Autodesk Fusion 360 part; units mm, degrees
(part 2 of 21)
sketch "Schizzo2" plane through (0, 0, 0) normal (0, 0, 1) x (1, 0, 0) in component "Spur Gear (12 teeth)"
  spline S0 degree 5 poles (5.5783, -0.8192) (5.5823, -0.8197) (5.5902, -0.8208) (5.6021, -0.8219) (5.6181, -0.8228) (5.6381, -0.8229) (5.6583, -0.8223) (5.6784, -0.8212) (5.6986, -0.8199) (5.7188, -0.8184) (5.7391, -0.8168) (5.7593, -0.8149) (5.7796, -0.8127) (5.7999, -0.8102) (5.8203, -0.8073) (5.8406, -0.8041) (5.861, -0.8006) (5.8814, -0.7969) (5.9018, -0.793) (5.9222, -0.7888) (5.9426, -0.7845) (5.9631, -0.7799) (5.9835, -0.7752) (6.0039, -0.7702) (6.0244, -0.765) (6.0448, -0.7596) (6.0653, -0.7539) (6.0857, -0.7481) (6.1061, -0.7421) (6.1266, -0.7359) (6.147, -0.7295) (6.1675, -0.7229) (6.1879, -0.7161) (6.2083, -0.7092) (6.2288, -0.7021) (6.2492, -0.6947) (6.2696, -0.6873) (6.29, -0.6796) (6.3104, -0.6717) (6.3308, -0.6637) (6.3512, -0.6555) (6.3715, -0.6472) (6.3919, -0.6387) (6.4122, -0.63) (6.4325, -0.6211) (6.4528, -0.6121) (6.4731, -0.6029) (6.4934, -0.5936) (6.5137, -0.5841) (6.5339, -0.5744) (6.5541, -0.5646) (6.5743, -0.5546) (6.5945, -0.5445) (6.6147, -0.5342) (6.6348, -0.5238) (6.655, -0.5132) (6.6751, -0.5024) (6.6951, -0.4915) (6.7152, -0.4805) (6.7352, -0.4693) (6.7552, -0.4579) (6.7752, -0.4464) (6.7952, -0.4348) (6.8151, -0.423) (6.835, -0.4111) (6.8549, -0.399) (6.8747, -0.3867) (6.8945, -0.3744) (6.9143, -0.3619) (6.9341, -0.3492) (6.9538, -0.3364) (6.9695, -0.3261) (6.9813, -0.3182) (6.9892, -0.313) (6.9931, -0.3103) knots 0 0 0 0 0 0 0.01428571 0.02857143 0.04285714 0.05714286 0.07142857 0.08571429 0.1 0.11428571 0.12857143 0.14285714 0.15714286 0.17142857 0.18571429 0.2 0.21428571 0.22857143 0.24285714 0.25714286 0.27142857 0.28571429 0.3 0.31428571 0.32857143 0.34285714 0.35714286 0.37142857 0.38571429 0.4 0.41428571 0.42857143 0.44285714 0.45714286 0.47142857 0.48571429 0.5 0.51428571 0.52857143 0.54285714 0.55714286 0.57142857 0.58571429 0.6 0.61428571 0.62857143 0.64285714 0.65714286 0.67142857 0.68571429 0.7 0.71428571 0.72857143 0.74285714 0.75714286 0.77142857 0.78571429 0.8 0.81428571 0.82857143 0.84285714 0.85714286 0.87142857 0.88571429 0.9 0.91428571 0.92857143 0.94285714 0.95714286 0.97142857 0.98571429 1 1 1 1 1 1
  spline S1 degree 5 poles (5.5783, 0.8192) (5.5823, 0.8197) (5.5902, 0.8208) (5.6021, 0.8219) (5.6181, 0.8228) (5.6381, 0.8229) (5.6583, 0.8223) (5.6784, 0.8212) (5.6986, 0.8199) (5.7188, 0.8184) (5.7391, 0.8168) (5.7593, 0.8149) (5.7796, 0.8127) (5.7999, 0.8102) (5.8203, 0.8073) (5.8406, 0.8041) (5.861, 0.8006) (5.8814, 0.7969) (5.9018, 0.793) (5.9222, 0.7888) (5.9426, 0.7845) (5.9631, 0.7799) (5.9835, 0.7752) (6.0039, 0.7702) (6.0244, 0.765) (6.0448, 0.7596) (6.0653, 0.7539) (6.0857, 0.7481) (6.1061, 0.7421) (6.1266, 0.7359) (6.147, 0.7295) (6.1675, 0.7229) (6.1879, 0.7161) (6.2083, 0.7092) (6.2288, 0.7021) (6.2492, 0.6947) (6.2696, 0.6873) (6.29, 0.6796) (6.3104, 0.6717) (6.3308, 0.6637) (6.3512, 0.6555) (6.3715, 0.6472) (6.3919, 0.6387) (6.4122, 0.63) (6.4325, 0.6211) (6.4528, 0.6121) (6.4731, 0.6029) (6.4934, 0.5936) (6.5137, 0.5841) (6.5339, 0.5744) (6.5541, 0.5646) (6.5743, 0.5546) (6.5945, 0.5445) (6.6147, 0.5342) (6.6348, 0.5238) (6.655, 0.5132) (6.6751, 0.5024) (6.6951, 0.4915) (6.7152, 0.4805) (6.7352, 0.4693) (6.7552, 0.4579) (6.7752, 0.4464) (6.7952, 0.4348) (6.8151, 0.423) (6.835, 0.4111) (6.8549, 0.399) (6.8747, 0.3867) (6.8945, 0.3744) (6.9143, 0.3619) (6.9341, 0.3492) (6.9538, 0.3364) (6.9695, 0.3261) (6.9813, 0.3182) (6.9892, 0.313) (6.9931, 0.3103) knots 0 0 0 0 0 0 0.01428571 0.02857143 0.04285714 0.05714286 0.07142857 0.08571429 0.1 0.11428571 0.12857143 0.14285714 0.15714286 0.17142857 0.18571429 0.2 0.21428571 0.22857143 0.24285714 0.25714286 0.27142857 0.28571429 0.3 0.31428571 0.32857143 0.34285714 0.35714286 0.37142857 0.38571429 0.4 0.41428571 0.42857143 0.44285714 0.45714286 0.47142857 0.48571429 0.5 0.51428571 0.52857143 0.54285714 0.55714286 0.57142857 0.58571429 0.6 0.61428571 0.62857143 0.64285714 0.65714286 0.67142857 0.68571429 0.7 0.71428571 0.72857143 0.74285714 0.75714286 0.77142857 0.78571429 0.8 0.81428571 0.82857143 0.84285714 0.85714286 0.87142857 0.88571429 0.9 0.91428571 0.92857143 0.94285714 0.95714286 0.97142857 0.98571429 1 1 1 1 1 1
  arc A0 (6.9931, -0.3103) -> (6.9931, 0.3103) centre (0, 0) ccw
  line L0 (4.6889, -0.69) -> (5.5783, -0.8192)
  line L1 (4.6889, 0.69) -> (5.5783, 0.8192)
  line L2 (4.6889, -0.69) -> (4.6889, 0.69)
  point P0 (5.6763, -0.8213)
  point P1 (5.7758, -0.8131)
  point P2 (5.8761, -0.7978)
  point P3 (5.977, -0.7767)
  point P4 (6.0784, -0.7502)
  point P5 (6.1802, -0.7187)
  point P6 (6.2821, -0.6825)
  point P7 (6.3842, -0.6419)
  point P8 (6.4862, -0.5969)
  point P9 (6.5882, -0.5477)
  point P10 (6.6899, -0.4943)
  point P11 (6.7914, -0.437)
  point P12 (6.8925, -0.3756)
  point P13 (5.6763, 0.8213)
  point P14 (5.7758, 0.8131)
  point P15 (5.8761, 0.7978)
  point P16 (5.977, 0.7767)
  point P17 (6.0784, 0.7502)
  point P18 (6.1802, 0.7187)
  point P19 (6.2821, 0.6825)
  point P20 (6.3842, 0.6419)
  point P21 (6.4862, 0.5969)
  point P22 (6.5882, 0.5477)
  point P23 (6.6899, 0.4943)
  point P24 (6.7914, 0.437)
  point P25 (6.8925, 0.3756)
extrude "Estrusione2" add sketch "Schizzo2" along normal blind 5 bodies 2 in component "Spur Gear (12 teeth)"
fillet "Raccordo1" radius 0.1 2 edges at (4.6986, -0.6914, 2.5) (4.6986, 0.6914, 2.5) on bodies 2 in component "Spur Gear (12 teeth)"
pattern_circular "Serie C1" count 12 over 360 about axis through (0, 0, 0) along (0, 0, 1) of "Estrusione2", "Raccordo1" in component "Spur Gear (12 teeth)"
sketch "Schizzo3" plane through (0, 0, 0) normal (0, 0, 1) x (1, 0, 0) in component "Spur Gear (12 teeth)"
  circle A0 centre (0, 0) radius 6 construction
combine "Combina1" operation add target body 1 tool bodies 2
extrude "Estrusione2'" cut 1 faces at (0.3611, -1.5413, 5) along direction (0, 0, -1) blind 1 on bodies 1 bodies 1
sketch "Schizzo2 (2)" plane through (0, 0, 4) normal (0, 0, 1) x (-1, 0, 0)
  arc A0 (-4.4499, 1.6593) -> (-4.6834, 0.788) centre (0, 0) ccw
  arc A1 (-4.7964, 0.7056) -> (-4.6834, 0.788) centre (-4.782, 0.8046) ccw
  line L0 (-4.7964, 0.7056) -> (-5.5783, 0.8192)
  spline S0 degree 3 poles (-6.9931, 0.3103) (-6.7925, 0.4447) (-6.5771, 0.5635) (-6.0115, 0.7938) (-5.7809, 0.814) (-5.6435, 0.8238) (-5.6102, 0.8238) (-5.5783, 0.8192) knots -0.02978 -0.02978 -0.02978 -0.02978 -0.021848 -0.021848 -0.009668 -0.009668 0 0 0 0
  arc A2 (-6.9931, 0.3103) -> (-6.9931, -0.3103) centre (0, 0) ccw
  spline S1 degree 3 poles (-5.5783, -0.8192) (-5.6911, -0.8355) (-5.8671, -0.8005) (-6.0076, -0.7707) (-6.1286, -0.7409) (-6.536, -0.586) (-6.7735, -0.4574) (-6.9931, -0.3103) knots -0.176502 -0.176502 -0.176502 -0.176502 -0.131302 -0.131302 -0.079288 -0.079288 0 0 0 0
  line L1 (-5.5783, -0.8192) -> (-4.7964, -0.7056)
  arc A3 (-4.6834, -0.788) -> (-4.7964, -0.7056) centre (-4.782, -0.8046) ccw
  arc A4 (-4.6834, -0.788) -> (-4.4499, -1.6593) centre (0, 0) ccw
  arc A5 (-4.5066, -1.7871) -> (-4.4499, -1.6593) centre (-4.5436, -1.6942) ccw
  line L2 (-4.5066, -1.7871) -> (-5.2406, -2.0798)
  spline S2 degree 3 poles (-6.2114, -3.2278) (-6.1048, -3.0111) (-5.9777, -2.8005) (-5.603, -2.3183) (-5.4134, -2.1855) (-5.2993, -2.1084) (-5.2705, -2.0917) (-5.2406, -2.0798) knots -0.02978 -0.02978 -0.02978 -0.02978 -0.021848 -0.021848 -0.009668 -0.009668 0 0 0 0
  arc A6 (-6.2114, -3.2278) -> (-5.901, -3.7653) centre (0, 0) ccw
  spline S3 degree 3 poles (-4.4214, -3.4986) (-4.5109, -3.5691) (-4.6808, -3.6268) (-4.8174, -3.6712) (-4.9371, -3.7059) (-5.3674, -3.7755) (-5.6373, -3.7829) (-5.901, -3.7653) knots -0.176502 -0.176502 -0.176502 -0.176502 -0.131302 -0.131302 -0.079288 -0.079288 0 0 0 0
  line L3 (-4.4214, -3.4986) -> (-3.801, -3.0093)
  arc A7 (-3.6619, -3.0241) -> (-3.801, -3.0093) centre (-3.739, -3.0878) ccw
  arc A8 (-3.6619, -3.0241) -> (-3.0241, -3.6619) centre (0, 0) ccw
  arc A9 (-3.0093, -3.801) -> (-3.0241, -3.6619) centre (-3.0878, -3.739) ccw
  line L4 (-3.0093, -3.801) -> (-3.4986, -4.4214)
  spline S4 degree 3 poles (-3.7653, -5.901) (-3.7814, -5.6601) (-3.7766, -5.4142) (-3.6932, -4.8092) (-3.5954, -4.5994) (-3.5352, -4.4756) (-3.5185, -4.4467) (-3.4986, -4.4214) knots -0.02978 -0.02978 -0.02978 -0.02978 -0.021848 -0.021848 -0.009668 -0.009668 0 0 0 0
  arc A10 (-3.7653, -5.901) -> (-3.2278, -6.2114) centre (0, 0) ccw
  spline S5 degree 3 poles (-2.0798, -5.2406) (-2.122, -5.3464) (-2.2403, -5.4813) (-2.3364, -5.5881) (-2.4227, -5.678) (-2.7605, -5.9534) (-2.9906, -6.0947) (-3.2278, -6.2114) knots -0.176502 -0.176502 -0.176502 -0.176502 -0.131302 -0.131302 -0.079288 -0.079288 0 0 0 0
  line L5 (-2.0798, -5.2406) -> (-1.7871, -4.5066)
  arc A11 (-1.6593, -4.4499) -> (-1.7871, -4.5066) centre (-1.6942, -4.5436) ccw
  arc A12 (-1.6593, -4.4499) -> (-0.788, -4.6834) centre (0, 0) ccw
  arc A13 (-0.7056, -4.7964) -> (-0.788, -4.6834) centre (-0.8046, -4.782) ccw
  line L6 (-0.7056, -4.7964) -> (-0.8192, -5.5783)
  spline S6 degree 3 poles (-0.3103, -6.9931) (-0.4447, -6.7925) (-0.5635, -6.5771) (-0.7938, -6.0115) (-0.814, -5.7809) (-0.8238, -5.6435) (-0.8238, -5.6102) (-0.8192, -5.5783) knots -0.02978 -0.02978 -0.02978 -0.02978 -0.021848 -0.021848 -0.009668 -0.009668 0 0 0 0
  arc A14 (-0.3103, -6.9931) -> (0.3103, -6.9931) centre (0, 0) ccw
  spline S7 degree 3 poles (0.8192, -5.5783) (0.8355, -5.6911) (0.8005, -5.8671) (0.7707, -6.0076) (0.7409, -6.1286) (0.586, -6.536) (0.4574, -6.7735) (0.3103, -6.9931) knots -0.176502 -0.176502 -0.176502 -0.176502 -0.131302 -0.131302 -0.079288 -0.079288 0 0 0 0
  line L7 (0.8192, -5.5783) -> (0.7056, -4.7964)
  arc A15 (0.788, -4.6834) -> (0.7056, -4.7964) centre (0.8046, -4.782) ccw
  arc A16 (0.788, -4.6834) -> (1.6593, -4.4499) centre (0, 0) ccw
  arc A17 (1.7871, -4.5066) -> (1.6593, -4.4499) centre (1.6942, -4.5436) ccw
  line L8 (1.7871, -4.5066) -> (2.0798, -5.2406)
  spline S8 degree 3 poles (3.2278, -6.2114) (3.0111, -6.1048) (2.8005, -5.9777) (2.3183, -5.603) (2.1855, -5.4134) (2.1084, -5.2993) (2.0917, -5.2705) (2.0798, -5.2406) knots -0.02978 -0.02978 -0.02978 -0.02978 -0.021848 -0.021848 -0.009668 -0.009668 0 0 0 0
  arc A18 (3.2278, -6.2114) -> (3.7653, -5.901) centre (0, 0) ccw
  spline S9 degree 3 poles (3.4986, -4.4214) (3.5691, -4.5109) (3.6268, -4.6808) (3.6712, -4.8174) (3.7059, -4.9371) (3.7755, -5.3674) (3.7829, -5.6373) (3.7653, -5.901) knots -0.176502 -0.176502 -0.176502 -0.176502 -0.131302 -0.131302 -0.079288 -0.079288 0 0 0 0
  line L9 (3.4986, -4.4214) -> (3.0093, -3.801)
  arc A19 (3.0241, -3.6619) -> (3.0093, -3.801) centre (3.0878, -3.739) ccw
  arc A20 (3.0241, -3.6619) -> (3.6619, -3.0241) centre (0, 0) ccw
  arc A21 (3.801, -3.0093) -> (3.6619, -3.0241) centre (3.739, -3.0878) ccw
  line L10 (3.801, -3.0093) -> (4.4214, -3.4986)
  spline S10 degree 3 poles (5.901, -3.7653) (5.6601, -3.7814) (5.4142, -3.7766) (4.8092, -3.6932) (4.5994, -3.5954) (4.4756, -3.5352) (4.4467, -3.5185) (4.4214, -3.4986) knots -0.02978 -0.02978 -0.02978 -0.02978 -0.021848 -0.021848 -0.009668 -0.009668 0 0 0 0
  arc A22 (5.901, -3.7653) -> (6.2114, -3.2278) centre (0, 0) ccw
  spline S11 degree 3 poles (5.2406, -2.0798) (5.3464, -2.122) (5.4813, -2.2403) (5.5881, -2.3364) (5.678, -2.4227) (5.9534, -2.7605) (6.0947, -2.9906) (6.2114, -3.2278) knots -0.176502 -0.176502 -0.176502 -0.176502 -0.131302 -0.131302 -0.079288 -0.079288 0 0 0 0
  line L11 (5.2406, -2.0798) -> (4.5066, -1.7871)
  arc A23 (4.4499, -1.6593) -> (4.5066, -1.7871) centre (4.5436, -1.6942) ccw
  arc A24 (4.4499, -1.6593) -> (4.6834, -0.788) centre (0, 0) ccw
  arc A25 (4.7964, -0.7056) -> (4.6834, -0.788) centre (4.782, -0.8046) ccw
  line L12 (4.7964, -0.7056) -> (5.5783, -0.8192)
  spline S12 degree 3 poles (6.9931, -0.3103) (6.7925, -0.4447) (6.5771, -0.5635) (6.0115, -0.7938) (5.7809, -0.814) (5.6435, -0.8238) (5.6102, -0.8238) (5.5783, -0.8192) knots -0.02978 -0.02978 -0.02978 -0.02978 -0.021848 -0.021848 -0.009668 -0.009668 0 0 0 0
  arc A26 (6.9931, -0.3103) -> (6.9931, 0.3103) centre (0, 0) ccw
  spline S13 degree 3 poles (5.5783, 0.8192) (5.6911, 0.8355) (5.8671, 0.8005) (6.0076, 0.7707) (6.1286, 0.7409) (6.536, 0.586) (6.7735, 0.4574) (6.9931, 0.3103) knots -0.176502 -0.176502 -0.176502 -0.176502 -0.131302 -0.131302 -0.079288 -0.079288 0 0 0 0
  line L13 (5.5783, 0.8192) -> (4.7964, 0.7056)
  arc A27 (4.6834, 0.788) -> (4.7964, 0.7056) centre (4.782, 0.8046) ccw
  arc A28 (4.6834, 0.788) -> (4.4499, 1.6593) centre (0, 0) ccw
  arc A29 (4.5066, 1.7871) -> (4.4499, 1.6593) centre (4.5436, 1.6942) ccw
  line L14 (4.5066, 1.7871) -> (5.2406, 2.0798)
  spline S14 degree 3 poles (6.2114, 3.2278) (6.1048, 3.0111) (5.9777, 2.8005) (5.603, 2.3183) (5.4134, 2.1855) (5.2993, 2.1084) (5.2705, 2.0917) (5.2406, 2.0798) knots -0.02978 -0.02978 -0.02978 -0.02978 -0.021848 -0.021848 -0.009668 -0.009668 0 0 0 0
  arc A30 (6.2114, 3.2278) -> (5.901, 3.7653) centre (0, 0) ccw
  spline S15 degree 3 poles (4.4214, 3.4986) (4.5109, 3.5691) (4.6808, 3.6268) (4.8174, 3.6712) (4.9371, 3.7059) (5.3674, 3.7755) (5.6373, 3.7829) (5.901, 3.7653) knots -0.176502 -0.176502 -0.176502 -0.176502 -0.131302 -0.131302 -0.079288 -0.079288 0 0 0 0
  line L15 (4.4214, 3.4986) -> (3.801, 3.0093)
  arc A31 (3.6619, 3.0241) -> (3.801, 3.0093) centre (3.739, 3.0878) ccw
  arc A32 (3.6619, 3.0241) -> (3.0241, 3.6619) centre (0, 0) ccw
  arc A33 (3.0093, 3.801) -> (3.0241, 3.6619) centre (3.0878, 3.739) ccw
  line L16 (3.0093, 3.801) -> (3.4986, 4.4214)
  spline S16 degree 3 poles (3.7653, 5.901) (3.7814, 5.6601) (3.7766, 5.4142) (3.6932, 4.8092) (3.5954, 4.5994) (3.5352, 4.4756) (3.5185, 4.4467) (3.4986, 4.4214) knots -0.02978 -0.02978 -0.02978 -0.02978 -0.021848 -0.021848 -0.009668 -0.009668 0 0 0 0
  arc A34 (3.7653, 5.901) -> (3.2278, 6.2114) centre (0, 0) ccw
  spline S17 degree 3 poles (2.0798, 5.2406) (2.122, 5.3464) (2.2403, 5.4813) (2.3364, 5.5881) (2.4227, 5.678) (2.7605, 5.9534) (2.9906, 6.0947) (3.2278, 6.2114) knots -0.176502 -0.176502 -0.176502 -0.176502 -0.131302 -0.131302 -0.079288 -0.079288 0 0 0 0
  line L17 (2.0798, 5.2406) -> (1.7871, 4.5066)
  arc A35 (1.6593, 4.4499) -> (1.7871, 4.5066) centre (1.6942, 4.5436) ccw
  arc A36 (1.6593, 4.4499) -> (0.788, 4.6834) centre (0, 0) ccw
  arc A37 (0.7056, 4.7964) -> (0.788, 4.6834) centre (0.8046, 4.782) ccw
  line L18 (0.7056, 4.7964) -> (0.8192, 5.5783)
  spline S18 degree 3 poles (0.3103, 6.9931) (0.4447, 6.7925) (0.5635, 6.5771) (0.7938, 6.0115) (0.814, 5.7809) (0.8238, 5.6435) (0.8238, 5.6102) (0.8192, 5.5783) knots -0.02978 -0.02978 -0.02978 -0.02978 -0.021848 -0.021848 -0.009668 -0.009668 0 0 0 0
  arc A38 (0.3103, 6.9931) -> (-0.3103, 6.9931) centre (0, 0) ccw
  spline S19 degree 3 poles (-0.8192, 5.5783) (-0.8355, 5.6911) (-0.8005, 5.8671) (-0.7707, 6.0076) (-0.7409, 6.1286) (-0.586, 6.536) (-0.4574, 6.7735) (-0.3103, 6.9931) knots -0.176502 -0.176502 -0.176502 -0.176502 -0.131302 -0.131302 -0.079288 -0.079288 0 0 0 0
  line L19 (-0.8192, 5.5783) -> (-0.7056, 4.7964)
  arc A39 (-0.788, 4.6834) -> (-0.7056, 4.7964) centre (-0.8046, 4.782) ccw
  arc A40 (-0.788, 4.6834) -> (-1.6593, 4.4499) centre (0, 0) ccw
  arc A41 (-1.7871, 4.5066) -> (-1.6593, 4.4499) centre (-1.6942, 4.5436) ccw
  line L20 (-1.7871, 4.5066) -> (-2.0798, 5.2406)
  spline S20 degree 3 poles (-3.2278, 6.2114) (-3.0111, 6.1048) (-2.8005, 5.9777) (-2.3183, 5.603) (-2.1855, 5.4134) (-2.1084, 5.2993) (-2.0917, 5.2705) (-2.0798, 5.2406) knots -0.02978 -0.02978 -0.02978 -0.02978 -0.021848 -0.021848 -0.009668 -0.009668 0 0 0 0
  arc A42 (-3.2278, 6.2114) -> (-3.7653, 5.901) centre (0, 0) ccw
  spline S21 degree 3 poles (-3.4986, 4.4214) (-3.5691, 4.5109) (-3.6268, 4.6808) (-3.6712, 4.8174) (-3.7059, 4.9371) (-3.7755, 5.3674) (-3.7829, 5.6373) (-3.7653, 5.901) knots -0.176502 -0.176502 -0.176502 -0.176502 -0.131302 -0.131302 -0.079288 -0.079288 0 0 0 0
  line L21 (-3.4986, 4.4214) -> (-3.0093, 3.801)
  arc A43 (-3.0241, 3.6619) -> (-3.0093, 3.801) centre (-3.0878, 3.739) ccw
  arc A44 (-3.0241, 3.6619) -> (-3.6619, 3.0241) centre (0, 0) ccw
  arc A45 (-3.801, 3.0093) -> (-3.6619, 3.0241) centre (-3.739, 3.0878) ccw
  line L22 (-3.801, 3.0093) -> (-4.4214, 3.4986)
  spline S22 degree 3 poles (-5.901, 3.7653) (-5.6601, 3.7814) (-5.4142, 3.7766) (-4.8092, 3.6932) (-4.5994, 3.5954) (-4.4756, 3.5352) (-4.4467, 3.5185) (-4.4214, 3.4986) knots -0.02978 -0.02978 -0.02978 -0.02978 -0.021848 -0.021848 -0.009668 -0.009668 0 0 0 0
  arc A46 (-5.901, 3.7653) -> (-6.2114, 3.2278) centre (0, 0) ccw
  spline S23 degree 3 poles (-5.2406, 2.0798) (-5.3464, 2.122) (-5.4813, 2.2403) (-5.5881, 2.3364) (-5.678, 2.4227) (-5.9534, 2.7605) (-6.0947, 2.9906) (-6.2114, 3.2278) knots -0.176502 -0.176502 -0.176502 -0.176502 -0.131302 -0.131302 -0.079288 -0.079288 0 0 0 0
  line L23 (-5.2406, 2.0798) -> (-4.5066, 1.7871)
  arc A47 (-4.4499, 1.6593) -> (-4.5066, 1.7871) centre (-4.5436, 1.6942) ccw
  circle A48 centre (0, 0) radius 4.7492
  circle A49 centre (0, 0) radius 3.1
  dimension "d14" = 9.4984
  dimension "d15" = 6.2
  constraint concentric A0 A48
  constraint concentric A48 A49
  measures "d14" diameter of A48
  measures "d15" diameter of A49
extrude "Estrusione3" add sketch "Schizzo2 (2)" along normal blind 5 contours A0 A4 A8 A12 A16 A20 A24 A28 A32 A36 A40 A44 A48 bodies 1
sketch "Schizzo3 (2)" plane through (0, 0, 0) normal (0, 0, -1) x (1, 0, 0)
  circle A0 centre (0, 0) radius 22.5
  circle A1 centre (3.1767, -12.1691) radius 2.7952
  line L0 (9.7097, -11.8871) -> (6.8258, -12.1397)
  line L1 (6.8258, -12.1397) -> (6.8538, -12.459)
  line L2 (6.8538, -12.459) -> (9.7377, -12.2064)
  line L3 (9.7377, -12.2064) -> (9.7097, -11.8871)
  line L4 (7.2966, -7.0628) -> (7.0295, -6.8856)
  line L5 (7.0295, -6.8856) -> (5.4289, -9.2978)
  line L6 (5.4289, -9.2978) -> (5.696, -9.475)
  line L7 (5.696, -9.475) -> (7.2966, -7.0628)
  line L8 (1.7531, -5.7644) -> (1.4481, -5.8627)
  line L9 (1.4481, -5.8627) -> (2.3361, -8.618)
  line L10 (2.3361, -8.618) -> (2.6412, -8.5197)
  line L11 (2.6412, -8.5197) -> (1.7531, -5.7644)
  line L12 (-2.7183, -9.2888) -> (-2.8316, -9.5887)
  line L13 (-2.8316, -9.5887) -> (-0.1237, -10.6123)
  line L14 (-0.1237, -10.6123) -> (-0.0104, -10.3125)
  line L15 (-0.0104, -10.3125) -> (-2.7183, -9.2888)
  line L16 (-2.7506, -14.9822) -> (-2.5869, -15.2577)
  line L17 (-2.5869, -15.2577) -> (-0.0983, -13.7789)
  line L18 (-0.0983, -13.7789) -> (-0.262, -13.5033)
  line L19 (-0.262, -13.5033) -> (-2.7506, -14.9822)
  line L20 (1.6804, -18.5572) -> (1.998, -18.601)
  line L21 (1.998, -18.601) -> (2.3934, -15.7333)
  line L22 (2.3934, -15.7333) -> (2.0758, -15.6895)
  line L23 (2.0758, -15.6895) -> (1.6804, -18.5572)
  line L24 (7.2383, -17.3219) -> (7.4705, -17.1009)
  line L25 (7.4705, -17.1009) -> (5.4749, -15.0038)
  line L26 (5.4749, -15.0038) -> (5.2427, -15.2247)
  line L27 (5.2427, -15.2247) -> (7.2383, -17.3219)
  circle A2 centre (-2.9782, 12.5602) radius 5.4022
  circle A3 centre (2.2614, 13.876) radius 7.9312
  circle A4 centre (-2.9782, 12.5602) radius 5.8068
  circle A5 centre (2.2614, 13.876) radius 7.4312
  line L28 (-4.3926, 18.1921) -> (-2.9782, 12.5602) construction
  line L29 (-2.9782, 12.5602) -> (-1.5637, 6.9282) construction
  dimension "d19" = 360
  dimension "d56" = -0.5
  constraint perpendicular L0 L1
  constraint parallel L0 L2
  constraint parallel L1 L3
  constraint concentric A2 A4
  constraint coincident A4 L28.start
  constraint coincident A2.centre A4.centre
  constraint coincident A4 L29.end
  constraint parallel L28 L29
  constraint coincident A3 L28.start
  constraint coincident A3 L29.end
  constraint coincident A2 A3.centre
extrude "Estrusione4" cut sketch "Schizzo3 (2)" against normal up to surface (1 mm away) contours A1 | L0 L1 L2 L3 | L4 L5 L6 L7 | L8 L9 L10 L11 | L12 L13 L14 L15 | L16 L17 L18 L19 | L20 L21 L22 L23 | L24 L25 L26 L27 | A2 A4 A5 | A2 A3 | A2 A3 A4 bodies 1
component "Spur Gear (12 teeth)" placed x (1, 0, 0) y (0, 1, 0) z (0, 0, 1) at (0, 0, 0)

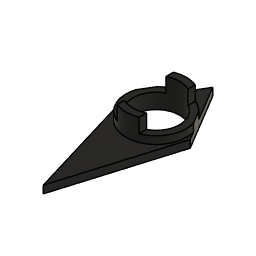
design "8 lancetta ore"
Autodesk Fusion 360 part; units mm, degrees
sketch "Schizzo1" plane through (0, 0, 0) normal (0, 0, 1) x (1, 0, 0)
  line L0 (0, -30) -> (9, 0)
  line L1 (9, 0) -> (0, 15)
  line L2 (0, 15) -> (-9, 0)
  line L3 (-9, 0) -> (0, -30)
  line L4 (0, -30) -> (0, 15) construction
  line L5 (9, 0) -> (-9, 0) construction
  circle A0 centre (0, 0) radius 6.2
  dimension "d1" = 30
  dimension "d2" = 15
  dimension "d3" = 9
  dimension "d12" = 12.4
  constraint vertical L4
  constraint perpendicular L4 L5
  constraint midpoint A0.centre L5
  constraint equal L0 L3
  constraint equal L1 L2
  constraint coincident A0.centre origin
  measures "d1" vertical distance of L0.start L0.end
  measures "d2" vertical distance of L0.end L1.end
  measures "d3" horizontal distance of L0.start L0.end
  measures "d12" diameter of A0
extrude "Estrusione1" add sketch "Schizzo1" along normal blind 2
sketch "Schizzo2" plane through (0, 0, 2) normal (0, 0, 1) x (-1, 0, 0)
  line L0 (9, 0) -> (0, 30)
  line L1 (0, 30) -> (-9, 0)
  line L2 (-9, 0) -> (0, -15)
  line L3 (0, -15) -> (9, 0)
  circle A0 centre (0, 0) radius 8
  circle A1 centre (0, 0) radius 6.2
  line L4 (-2.9, 24) -> (2.9, 24)
  line L5 (2.9, 24) -> (2.9, -21)
  line L6 (2.9, -21) -> (-2.9, -21)
  line L7 (-2.9, -21) -> (-2.9, 24)
  circle A2 centre (0, 0) radius 6.2
  dimension "d6" = 16
  dimension "d7" = 12.4
  dimension "d8" = 2.9
  dimension "d9" = 2.9
  constraint coincident A0.centre A1.centre
  constraint horizontal L4
  constraint vertical L5
  constraint horizontal L6
  constraint vertical L7
  measures "d6" diameter of A0
  measures "d7" diameter of A1
  measures "d8" distance of A0.centre L7
  measures "d9" distance of A0.centre L5
extrude "Estrusione2" add sketch "Schizzo2" along normal blind 5.8 contours A0 A1 L5 L7 A2 | A0 A1 L5 L7 A2
sketch "Schizzo3" plane through (0, 0, 2) normal (0, 0, 1) x (-1, 0, 0)
  line L0 (9, 0) -> (0, 30)
  line L1 (0, 30) -> (-9, 0)
  line L2 (-9, 0) -> (0, -15)
  line L3 (0, -15) -> (9, 0)
  circle A0 centre (0, 0) radius 8
  circle A1 centre (0, 0) radius 6.2
  arc A2 (2.9, -5.48) -> (2.9, 5.48) centre (0, 0) ccw
  arc A3 (2.9, 5.48) -> (-2.9, 5.48) centre (0, 0) ccw
  line L4 (-2.9, 5.48) -> (-2.9, 7.4559)
  arc A4 (2.9, 7.4559) -> (-2.9, 7.4559) centre (0, 0) ccw
  line L5 (2.9, 7.4559) -> (2.9, 5.48)
  line L6 (2.9, -5.48) -> (2.9, -7.4559)
  arc A5 (-2.9, -7.4559) -> (2.9, -7.4559) centre (0, 0) ccw
  line L7 (-2.9, -7.4559) -> (-2.9, -5.48)
  arc A6 (-2.9, 5.48) -> (-2.9, -5.48) centre (0, 0) ccw
  line L8 (2.9, -5.48) -> (2.9, -7.4559)
  arc A7 (-2.9, -7.4559) -> (2.9, -7.4559) centre (0, 0) ccw
  line L9 (-2.9, -7.4559) -> (-2.9, -5.48)
  arc A8 (-2.9, 5.48) -> (-2.9, -5.48) centre (0, 0) ccw
  line L10 (-2.9, 5.48) -> (-2.9, 7.4559)
  arc A9 (2.9, 7.4559) -> (-2.9, 7.4559) centre (0, 0) ccw
  line L11 (2.9, 7.4559) -> (2.9, 5.48)
  arc A10 (2.9, -5.48) -> (2.9, 5.48) centre (0, 0) ccw
  line L12 (9, 0) -> (0, 30)
  line L13 (0, 30) -> (-9, 0)
  line L14 (-9, 0) -> (0, -15)
  line L15 (0, -15) -> (9, 0)
  dimension "d15" = 16
  constraint concentric A0 A1
  constraint concentric A1 A3
  constraint equal A1 A3
  measures "d15" diameter of A0
extrude "Estrusione3" add sketch "Schizzo3" along normal blind 2 contours L3 A0 A1 A2 L5 L6 L8 L11 A10 L15 | L2 A0 A1 L4 L7 A6 L9 A8 L10 L14 | A0 A1 L6 A5 L7 L8 A7 L9 | A0 A1 A3 L4 A4 L5 L10 A9 L11

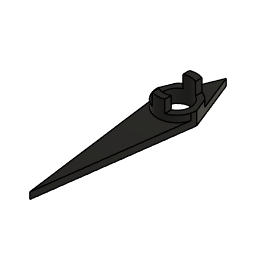
design "5 lancetta minuti"
Autodesk Fusion 360 part; units mm, degrees
sketch "Schizzo1" plane through (0, 0, 0) normal (0, 0, 1) x (1, 0, 0)
  line L0 (0, -45) -> (6, 0)
  line L1 (6, 0) -> (0, 15)
  line L2 (0, 15) -> (-6, 0)
  line L3 (-6, 0) -> (0, -45)
  line L4 (0, -45) -> (0, 15) construction
  line L5 (6, 0) -> (-6, 0) construction
  circle A0 centre (0, 0) radius 4.15
  circle A1 centre (0, 0) radius 6 construction
  dimension "d1" = 45
  dimension "d2" = 15
  dimension "d3" = 6
  dimension "d12" = 8.3
  dimension "d15" = 12
  constraint vertical L4
  constraint perpendicular L4 L5
  constraint midpoint A0.centre L5
  constraint equal L0 L3
  constraint equal L1 L2
  constraint coincident A0.centre A1.centre
  measures "d1" vertical distance of L0.start L0.end
  measures "d2" vertical distance of L0.end L1.end
  measures "d3" horizontal distance of L0.start L0.end
  measures "d12" diameter of A0
  measures "d15" diameter of A1
extrude "Estrusione1" add sketch "Schizzo1" along normal blind 2
sketch "Schizzo2" plane through (0, 0, 2) normal (0, 0, 1) x (-1, 0, 0)
  line L0 (6, 0) -> (0, 45)
  line L1 (0, 45) -> (-6, 0)
  line L2 (-6, 0) -> (0, -15)
  line L3 (0, -15) -> (6, 0)
  circle A0 centre (0, 0) radius 6
  circle A1 centre (0, 0) radius 4.15
  line L4 (-1.9, 24) -> (1.9, 24)
  line L5 (1.9, 24) -> (1.9, -21)
  line L6 (1.9, -21) -> (-1.9, -21)
  line L7 (-1.9, -21) -> (-1.9, 24)
  circle A2 centre (0, 0) radius 4.15
  circle A3 centre (0, 0) radius 4.15
  line L8 (6, 0) -> (0, 45)
  line L9 (0, 45) -> (-6, 0)
  line L10 (-6, 0) -> (0, -15)
  line L11 (0, -15) -> (6, 0)
  dimension "d6" = 12
  dimension "d7" = 8.3
  dimension "d8" = 1.9
  dimension "d9" = 1.9
  constraint coincident A0.centre A1.centre
  constraint horizontal L4
  constraint vertical L5
  constraint horizontal L6
  constraint vertical L7
  measures "d6" diameter of A0
  measures "d7" diameter of A1
  measures "d8" distance of A0.centre L7
  measures "d9" distance of A0.centre L5
extrude "Estrusione2" add sketch "Schizzo2" along normal blind 5.8 contours A0 A1 L5 L7 A2 A3 | A0 A1 L5 L7 A2 A3
sketch "Schizzo3" plane through (0, 0, 2) normal (0, 0, 1) x (-1, 0, 0)
  line L0 (-1.9, 3.6895) -> (-1.9, 5.6912)
  arc A0 (1.9, 5.6912) -> (-1.9, 5.6912) centre (0, 0) ccw
  line L1 (1.9, 5.6912) -> (1.9, 3.6895)
  arc A1 (1.9, -3.6895) -> (1.9, 3.6895) centre (0, 0) ccw
  line L2 (1.9, -3.6895) -> (1.9, -5.6912)
  arc A2 (-1.9, -5.6912) -> (1.9, -5.6912) centre (0, 0) ccw
  line L3 (-1.9, -5.6912) -> (-1.9, -3.6895)
  arc A3 (-1.9, 3.6895) -> (-1.9, -3.6895) centre (0, 0) ccw
  line L4 (6, 0) -> (0, 45)
  line L5 (0, 45) -> (-6, 0)
  line L6 (-6, 0) -> (0, -15)
  line L7 (0, -15) -> (6, 0)
  circle A4 centre (0, 0) radius 4.15
  circle A5 centre (0, 0) radius 6
  constraint concentric A0 A4
  constraint coincident L3.end A4
  constraint concentric A4 A5
  constraint coincident A2.start A5
extrude "Estrusione3" add sketch "Schizzo3" along normal blind 2 contours L0 L3 A3 L5 L6 A4 A5 | L1 A1 L2 L4 L7 A4 A5

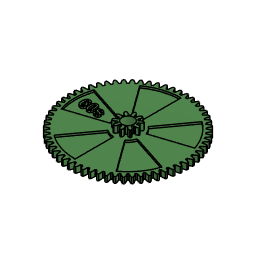
design "3 intermedio minuti"
description: Spur Gear; Module: 1.000000; Num Teeth: 60; Pressure Angle: 20.000000; Backlash: 0.00 mm
description: Spur Gear; Module: 1.000000; Num Teeth: 10; Pressure Angle: 20.000000; Backlash: 0.00 mm
Autodesk Fusion 360 part; units mm, degrees
sketch "Schizzo1" plane through (0, 0, 0) normal (0, 0, 1) x (1, 0, 0) in component "Spur Gear (60 teeth)"
  circle A0 centre (0, 0) radius 28.7492
  circle A1 centre (0, 0) radius 3.1
extrude "Estrusione1" add sketch "Schizzo1" along normal blind 3 makes body 1 in component "Spur Gear (60 teeth)"
sketch "Schizzo2" plane through (0, 0, 0) normal (0, 0, 1) x (1, 0, 0) in component "Spur Gear (60 teeth)"
  spline S0 degree 5 poles (28.167, -1.1579) (28.1751, -1.1579) (28.1914, -1.1578) (28.2159, -1.1575) (28.2485, -1.1567) (28.2892, -1.1551) (28.33, -1.1529) (28.3707, -1.1501) (28.4115, -1.1467) (28.4523, -1.1427) (28.493, -1.1383) (28.5338, -1.1335) (28.5746, -1.1284) (28.6154, -1.1228) (28.6561, -1.117) (28.6969, -1.1109) (28.7376, -1.1045) (28.7783, -1.0977) (28.8191, -1.0907) (28.8598, -1.0834) (28.9005, -1.0758) (28.9412, -1.0679) (28.9819, -1.0597) (29.0226, -1.0513) (29.0633, -1.0427) (29.104, -1.0338) (29.1446, -1.0247) (29.1853, -1.0153) (29.2259, -1.0057) (29.2665, -0.9959) (29.3071, -0.9858) (29.3477, -0.9755) (29.3883, -0.965) (29.4289, -0.9543) (29.4694, -0.9434) (29.5099, -0.9323) (29.5505, -0.921) (29.591, -0.9094) (29.6315, -0.8977) (29.672, -0.8858) (29.7124, -0.8737) (29.7529, -0.8614) (29.7933, -0.8488) (29.8337, -0.8361) (29.8741, -0.8233) (29.9145, -0.8102) (29.9549, -0.7969) (29.9952, -0.7835) (30.0355, -0.7699) (30.0759, -0.7561) (30.1161, -0.7421) (30.1564, -0.728) (30.1967, -0.7137) (30.2369, -0.6992) (30.2771, -0.6845) (30.3173, -0.6697) (30.3575, -0.6547) (30.3977, -0.6396) (30.4378, -0.6242) (30.4779, -0.6087) (30.518, -0.5931) (30.5581, -0.5773) (30.5982, -0.5613) (30.6382, -0.5451) (30.6782, -0.5288) (30.7182, -0.5124) (30.7582, -0.4958) (30.7981, -0.479) (30.838, -0.4621) (30.8779, -0.445) (30.9178, -0.4278) (30.9497, -0.4139) (30.9736, -0.4034) (30.9895, -0.3963) (30.9975, -0.3928) knots 0 0 0 0 0 0 0.01428571 0.02857143 0.04285714 0.05714286 0.07142857 0.08571429 0.1 0.11428571 0.12857143 0.14285714 0.15714286 0.17142857 0.18571429 0.2 0.21428571 0.22857143 0.24285714 0.25714286 0.27142857 0.28571429 0.3 0.31428571 0.32857143 0.34285714 0.35714286 0.37142857 0.38571429 0.4 0.41428571 0.42857143 0.44285714 0.45714286 0.47142857 0.48571429 0.5 0.51428571 0.52857143 0.54285714 0.55714286 0.57142857 0.58571429 0.6 0.61428571 0.62857143 0.64285714 0.65714286 0.67142857 0.68571429 0.7 0.71428571 0.72857143 0.74285714 0.75714286 0.77142857 0.78571429 0.8 0.81428571 0.82857143 0.84285714 0.85714286 0.87142857 0.88571429 0.9 0.91428571 0.92857143 0.94285714 0.95714286 0.97142857 0.98571429 1 1 1 1 1 1
  spline S1 degree 5 poles (28.167, 1.1579) (28.1751, 1.1579) (28.1914, 1.1578) (28.2159, 1.1575) (28.2485, 1.1567) (28.2892, 1.1551) (28.33, 1.1529) (28.3707, 1.1501) (28.4115, 1.1467) (28.4523, 1.1427) (28.493, 1.1383) (28.5338, 1.1335) (28.5746, 1.1284) (28.6154, 1.1228) (28.6561, 1.117) (28.6969, 1.1109) (28.7376, 1.1045) (28.7783, 1.0977) (28.8191, 1.0907) (28.8598, 1.0834) (28.9005, 1.0758) (28.9412, 1.0679) (28.9819, 1.0597) (29.0226, 1.0513) (29.0633, 1.0427) (29.104, 1.0338) (29.1446, 1.0247) (29.1853, 1.0153) (29.2259, 1.0057) (29.2665, 0.9959) (29.3071, 0.9858) (29.3477, 0.9755) (29.3883, 0.965) (29.4289, 0.9543) (29.4694, 0.9434) (29.5099, 0.9323) (29.5505, 0.921) (29.591, 0.9094) (29.6315, 0.8977) (29.672, 0.8858) (29.7124, 0.8737) (29.7529, 0.8614) (29.7933, 0.8488) (29.8337, 0.8361) (29.8741, 0.8233) (29.9145, 0.8102) (29.9549, 0.7969) (29.9952, 0.7835) (30.0355, 0.7699) (30.0759, 0.7561) (30.1161, 0.7421) (30.1564, 0.728) (30.1967, 0.7137) (30.2369, 0.6992) (30.2771, 0.6845) (30.3173, 0.6697) (30.3575, 0.6547) (30.3977, 0.6396) (30.4378, 0.6242) (30.4779, 0.6087) (30.518, 0.5931) (30.5581, 0.5773) (30.5982, 0.5613) (30.6382, 0.5451) (30.6782, 0.5288) (30.7182, 0.5124) (30.7582, 0.4958) (30.7981, 0.479) (30.838, 0.4621) (30.8779, 0.445) (30.9178, 0.4278) (30.9497, 0.4139) (30.9736, 0.4034) (30.9895, 0.3963) (30.9975, 0.3928) knots 0 0 0 0 0 0 0.01428571 0.02857143 0.04285714 0.05714286 0.07142857 0.08571429 0.1 0.11428571 0.12857143 0.14285714 0.15714286 0.17142857 0.18571429 0.2 0.21428571 0.22857143 0.24285714 0.25714286 0.27142857 0.28571429 0.3 0.31428571 0.32857143 0.34285714 0.35714286 0.37142857 0.38571429 0.4 0.41428571 0.42857143 0.44285714 0.45714286 0.47142857 0.48571429 0.5 0.51428571 0.52857143 0.54285714 0.55714286 0.57142857 0.58571429 0.6 0.61428571 0.62857143 0.64285714 0.65714286 0.67142857 0.68571429 0.7 0.71428571 0.72857143 0.74285714 0.75714286 0.77142857 0.78571429 0.8 0.81428571 0.82857143 0.84285714 0.85714286 0.87142857 0.88571429 0.9 0.91428571 0.92857143 0.94285714 0.95714286 0.97142857 0.98571429 1 1 1 1 1 1
  arc A0 (30.9975, -0.3928) -> (30.9975, 0.3928) centre (0, 0) ccw
  line L0 (28.167, 1.1579) -> (28.167, -1.1579)
  point P0 (28.3681, -1.1501)
  point P1 (28.5698, -1.1289)
  point P2 (28.7718, -1.0988)
  point P3 (28.974, -1.0613)
  point P4 (29.1763, -1.0173)
  point P5 (29.3788, -0.9675)
  point P6 (29.5813, -0.9122)
  point P7 (29.7839, -0.8517)
  point P8 (29.9864, -0.7864)
  point P9 (30.1889, -0.7164)
  point P10 (30.3912, -0.6419)
  point P11 (30.5935, -0.5631)
  point P12 (30.7956, -0.48)
  point P13 (28.3681, 1.1501)
  point P14 (28.5698, 1.1289)
  point P15 (28.7718, 1.0988)
  point P16 (28.974, 1.0613)
  point P17 (29.1763, 1.0173)
  point P18 (29.3788, 0.9675)
  point P19 (29.5813, 0.9122)
  point P20 (29.7839, 0.8517)
  point P21 (29.9864, 0.7864)
  point P22 (30.1889, 0.7164)
  point P23 (30.3912, 0.6419)
  point P24 (30.5935, 0.5631)
  point P25 (30.7956, 0.48)
extrude "Estrusione2" add sketch "Schizzo2" along normal blind 3 bodies 1 in component "Spur Gear (60 teeth)"
fillet "Raccordo1" radius 0.1 2 edges at (28.7279, 1.1059, 1.5) (28.7279, -1.1059, 1.5) on bodies 1 in component "Spur Gear (60 teeth)"
pattern_circular "Serie C1" count 60 over 360 about axis through (0, 0, 0) along (0, 0, 1) of "Estrusione2", "Raccordo1" in component "Spur Gear (60 teeth)"
sketch "Schizzo3" plane through (0, 0, 0) normal (0, 0, 1) x (1, 0, 0) in component "Spur Gear (60 teeth)"
  circle A0 centre (0, 0) radius 30 construction
sketch "Schizzo1 (2)" plane through (0, 0, 0) normal (0, 0, 1) x (1, 0, 0) in component "Spur Gear (10 teeth)"
  circle A0 centre (0, 0) radius 3.7492
  circle A1 centre (0, 0) radius 3.1
extrude "Estrusione1'" add sketch "Schizzo1 (2)" along normal blind 3 separate body makes body 2 in component "Spur Gear (10 teeth)"
sketch "Schizzo2 (2)" plane through (0, 0, 0) normal (0, 0, 1) x (1, 0, 0) in component "Spur Gear (10 teeth)"
  spline S0 degree 5 poles (4.6291, -0.8041) (4.6329, -0.8047) (4.6405, -0.8059) (4.6519, -0.8073) (4.6672, -0.8084) (4.6864, -0.8088) (4.7057, -0.8085) (4.7251, -0.8077) (4.7445, -0.8066) (4.7639, -0.8054) (4.7834, -0.804) (4.8029, -0.8024) (4.8224, -0.8004) (4.842, -0.7981) (4.8616, -0.7954) (4.8812, -0.7924) (4.9009, -0.7891) (4.9205, -0.7856) (4.9402, -0.7818) (4.9599, -0.7778) (4.9796, -0.7737) (4.9993, -0.7693) (5.019, -0.7646) (5.0388, -0.7598) (5.0585, -0.7547) (5.0783, -0.7493) (5.098, -0.7438) (5.1178, -0.738) (5.1375, -0.7321) (5.1573, -0.7259) (5.177, -0.7196) (5.1968, -0.7131) (5.2165, -0.7063) (5.2363, -0.6994) (5.256, -0.6923) (5.2757, -0.685) (5.2955, -0.6775) (5.3152, -0.6698) (5.3349, -0.6619) (5.3546, -0.6538) (5.3743, -0.6456) (5.394, -0.6372) (5.4136, -0.6286) (5.4333, -0.6198) (5.4529, -0.6109) (5.4725, -0.6018) (5.4921, -0.5925) (5.5117, -0.583) (5.5312, -0.5734) (5.5508, -0.5636) (5.5703, -0.5536) (5.5898, -0.5435) (5.6093, -0.5332) (5.6287, -0.5228) (5.6482, -0.5121) (5.6676, -0.5013) (5.6869, -0.4904) (5.7063, -0.4793) (5.7256, -0.468) (5.7449, -0.4566) (5.7642, -0.445) (5.7834, -0.4332) (5.8026, -0.4213) (5.8218, -0.4093) (5.8409, -0.397) (5.86, -0.3847) (5.8791, -0.3721) (5.8982, -0.3595) (5.9172, -0.3466) (5.9361, -0.3336) (5.9551, -0.3205) (5.9702, -0.3099) (5.9815, -0.3018) (5.989, -0.2964) (5.9928, -0.2937) knots 0 0 0 0 0 0 0.01428571 0.02857143 0.04285714 0.05714286 0.07142857 0.08571429 0.1 0.11428571 0.12857143 0.14285714 0.15714286 0.17142857 0.18571429 0.2 0.21428571 0.22857143 0.24285714 0.25714286 0.27142857 0.28571429 0.3 0.31428571 0.32857143 0.34285714 0.35714286 0.37142857 0.38571429 0.4 0.41428571 0.42857143 0.44285714 0.45714286 0.47142857 0.48571429 0.5 0.51428571 0.52857143 0.54285714 0.55714286 0.57142857 0.58571429 0.6 0.61428571 0.62857143 0.64285714 0.65714286 0.67142857 0.68571429 0.7 0.71428571 0.72857143 0.74285714 0.75714286 0.77142857 0.78571429 0.8 0.81428571 0.82857143 0.84285714 0.85714286 0.87142857 0.88571429 0.9 0.91428571 0.92857143 0.94285714 0.95714286 0.97142857 0.98571429 1 1 1 1 1 1
  spline S1 degree 5 poles (4.6291, 0.8041) (4.6329, 0.8047) (4.6405, 0.8059) (4.6519, 0.8073) (4.6672, 0.8084) (4.6864, 0.8088) (4.7057, 0.8085) (4.7251, 0.8077) (4.7445, 0.8066) (4.7639, 0.8054) (4.7834, 0.804) (4.8029, 0.8024) (4.8224, 0.8004) (4.842, 0.7981) (4.8616, 0.7954) (4.8812, 0.7924) (4.9009, 0.7891) (4.9205, 0.7856) (4.9402, 0.7818) (4.9599, 0.7778) (4.9796, 0.7737) (4.9993, 0.7693) (5.019, 0.7646) (5.0388, 0.7598) (5.0585, 0.7547) (5.0783, 0.7493) (5.098, 0.7438) (5.1178, 0.738) (5.1375, 0.7321) (5.1573, 0.7259) (5.177, 0.7196) (5.1968, 0.7131) (5.2165, 0.7063) (5.2363, 0.6994) (5.256, 0.6923) (5.2757, 0.685) (5.2955, 0.6775) (5.3152, 0.6698) (5.3349, 0.6619) (5.3546, 0.6538) (5.3743, 0.6456) (5.394, 0.6372) (5.4136, 0.6286) (5.4333, 0.6198) (5.4529, 0.6109) (5.4725, 0.6018) (5.4921, 0.5925) (5.5117, 0.583) (5.5312, 0.5734) (5.5508, 0.5636) (5.5703, 0.5536) (5.5898, 0.5435) (5.6093, 0.5332) (5.6287, 0.5228) (5.6482, 0.5121) (5.6676, 0.5013) (5.6869, 0.4904) (5.7063, 0.4793) (5.7256, 0.468) (5.7449, 0.4566) (5.7642, 0.445) (5.7834, 0.4332) (5.8026, 0.4213) (5.8218, 0.4093) (5.8409, 0.397) (5.86, 0.3847) (5.8791, 0.3721) (5.8982, 0.3595) (5.9172, 0.3466) (5.9361, 0.3336) (5.9551, 0.3205) (5.9702, 0.3099) (5.9815, 0.3018) (5.989, 0.2964) (5.9928, 0.2937) knots 0 0 0 0 0 0 0.01428571 0.02857143 0.04285714 0.05714286 0.07142857 0.08571429 0.1 0.11428571 0.12857143 0.14285714 0.15714286 0.17142857 0.18571429 0.2 0.21428571 0.22857143 0.24285714 0.25714286 0.27142857 0.28571429 0.3 0.31428571 0.32857143 0.34285714 0.35714286 0.37142857 0.38571429 0.4 0.41428571 0.42857143 0.44285714 0.45714286 0.47142857 0.48571429 0.5 0.51428571 0.52857143 0.54285714 0.55714286 0.57142857 0.58571429 0.6 0.61428571 0.62857143 0.64285714 0.65714286 0.67142857 0.68571429 0.7 0.71428571 0.72857143 0.74285714 0.75714286 0.77142857 0.78571429 0.8 0.81428571 0.82857143 0.84285714 0.85714286 0.87142857 0.88571429 0.9 0.91428571 0.92857143 0.94285714 0.95714286 0.97142857 0.98571429 1 1 1 1 1 1
  arc A0 (5.9928, -0.2937) -> (5.9928, 0.2937) centre (0, 0) ccw
  line L0 (3.684, -0.6416) -> (4.6291, -0.8041)
  line L1 (3.684, 0.6416) -> (4.6291, 0.8041)
  line L2 (3.684, -0.6416) -> (3.684, 0.6416)
  point P0 (4.7229, -0.8077)
  point P1 (4.8183, -0.8008)
  point P2 (4.9148, -0.7866)
  point P3 (5.0121, -0.7662)
  point P4 (5.11, -0.7403)
  point P5 (5.2082, -0.7091)
  point P6 (5.3067, -0.673)
  point P7 (5.4054, -0.6322)
  point P8 (5.504, -0.5867)
  point P9 (5.6025, -0.5368)
  point P10 (5.7007, -0.4824)
  point P11 (5.7986, -0.4238)
  point P12 (5.896, -0.3609)
  point P13 (4.7229, 0.8077)
  point P14 (4.8183, 0.8008)
  point P15 (4.9148, 0.7866)
  point P16 (5.0121, 0.7662)
  point P17 (5.11, 0.7403)
  point P18 (5.2082, 0.7091)
  point P19 (5.3067, 0.673)
  point P20 (5.4054, 0.6322)
  point P21 (5.504, 0.5867)
  point P22 (5.6025, 0.5368)
  point P23 (5.7007, 0.4824)
  point P24 (5.7986, 0.4238)
  point P25 (5.896, 0.3609)
extrude "Estrusione2'" add sketch "Schizzo2 (2)" along normal blind 3 bodies 2 in component "Spur Gear (10 teeth)"
fillet "Raccordo1'" radius 0.1 2 edges at (3.6936, -0.6433, 1.5) (3.6936, 0.6433, 1.5) on bodies 2 in component "Spur Gear (10 teeth)"
pattern_circular "Serie C1'" count 10 over 360 about axis through (0, 0, 0) along (0, 0, 1) of "Estrusione2'", "Raccordo1'" in component "Spur Gear (10 teeth)"
sketch "Schizzo3 (2)" plane through (0, 0, 0) normal (0, 0, 1) x (1, 0, 0) in component "Spur Gear (10 teeth)"
  circle A0 centre (0, 0) radius 5 construction
move_body "Sposta1" bodies 2 to x (1, 0, 0) y (0, 1, 0) z (0, 0, 1) at (0, 0, 3) in component "Spur Gear (10 teeth)"
combine "Combina1" operation add target body 1 tool bodies 2 in component "Spur Gear (60 teeth)"
extrude "Estrusione3" add 1 faces at (-3.6482, -2.3787, 6) along direction (0, 0, 1) blind 2 on bodies 1 bodies 1 in component "Spur Gear (60 teeth)"